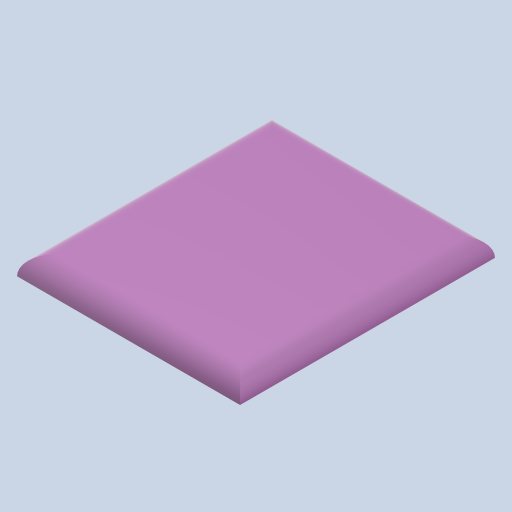
# Autodesk Inventor part: Part6
Saved by Autodesk Inventor 2024 (Build 280153000, 153)
## iProperties
Created: 2024-05-29
Part Number: Part6
Material: Generic
Document SubType Name: Modeling
Designer: mirun
Density: 1 g/cm^3
Appearance: Smooth - Purple
Author: mirun
Autodesk Inventor part; units mm, degrees
ref_plane "YZ Plane" through (0, 0, 0) normal (1, 0, 0) x (0, 1, 0)
ref_plane "XZ Plane" through (0, 0, 0) normal (0, 1, 0) x (-1, 0, 0)
ref_plane "XY Plane" through (0, 0, 0) normal (0, 0, 1) x (1, 0, 0)
sketch "Sketch1" plane through (0, 0, 0) normal (0, 1, 0) x (-1, 0, 0)
  line L0 (-175, 200) -> (175, 200)
  line L1 (175, 200) -> (175, -200)
  line L2 (175, -200) -> (-175, -200)
  line L3 (-175, -200) -> (-175, 200)
  line L4 (-175, 200) -> (175, -200) construction
  line L5 (175, 200) -> (-175, -200) construction
  point P0 (0, 0)
  dimension "d0" = 350
  dimension "d1" = 400
  constraints: 12 end point, 2 midpoint, 2 parallel, 1 horizontal, 1 perpendicular
  measures "d0" distance of L0.start L0.end
  measures "d1" distance of L0.end L1.end
extrude "Extrusion1" add sketch "Sketch1" along normal blind 30
fillet "Fillet1" radius 30 4 edges at (0, 30, 200) (-175, 30, 0) (175, 30, 0) (0, 30, -200)
body "Solid1"
